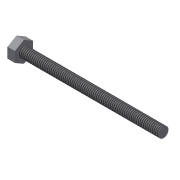
# Autodesk Inventor part: Šrouv M12x160
Saved by Autodesk Inventor 2015 (Build 190159000, 159)
## iProperties
Created: 2015-01-09
Part Number: Šrouv M12x160
Material: Všeobecné
Document SubType Name: Modeling
Designer: Michal
Density: 1 g/cm^3
Appearance: Výchozí
Author: Michal
Autodesk Inventor part; units mm, degrees
ref_plane "YZ Plane" through (0, 0, 0) normal (1, 0, 0) x (0, 1, 0)
ref_plane "XZ Plane" through (0, 0, 0) normal (0, 1, 0) x (-1, 0, 0)
ref_plane "XY Plane" through (0, 0, 0) normal (0, 0, 1) x (1, 0, 0)
sketch "Náčrt1" plane through (0, 0, 0) normal (1, 0, 0) x (0, 1, 0)
  line L0 (0, -10.3923) -> (-9, -5.1962)
  line L1 (-9, -5.1962) -> (-9, 5.1962)
  line L2 (-9, 5.1962) -> (0, 10.3923)
  line L3 (0, 10.3923) -> (9, 5.1962)
  line L4 (9, 5.1962) -> (9, -5.1962)
  line L5 (9, -5.1962) -> (0, -10.3923)
  point P0 (0, 0)
  point P1 (0, 0)
  dimension "d0" = 18
  constraints: 12 end point, 1 coincident, 13 other
  measures "d0" distance between parallel lines of L5 L2
extrude "Vysunutí1" add sketch "Náčrt1" along normal blind 7.5
sketch "Náčrt2" plane through (7.5, 0, 0) normal (1, 0, 0) x (0, 0, -1)
  circle A0 centre (0, 0) radius 5
  dimension "d3" = 10
  constraints: 1 centre point, 1 coincident
  measures "d3" diameter of A0
extrude "Vysunutí2" add sketch "Náčrt2" along normal blind 140
thread "Závit1" size "M12x1.75" class "6g" standard "ANSI Metric M Profile" full length
